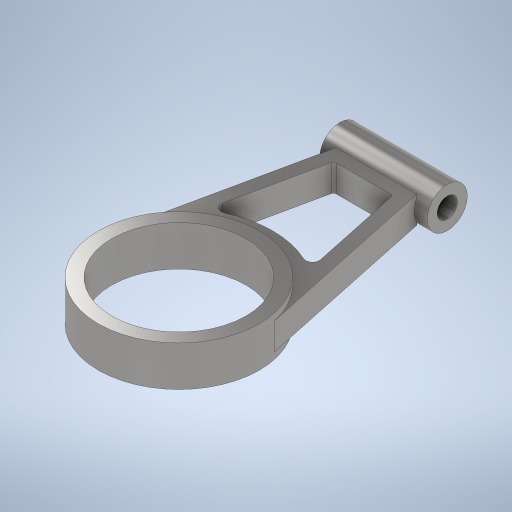
# Autodesk Inventor part: Excercise4
Saved by Autodesk Inventor 2024 (Build 280153000, 153)
## iProperties
Created: 2024-03-22
Part Number: Excercise4
Material: Stahl, galvanisiert
Document SubType Name: Modeling
Designer: ffogue
Density: 7.85 g/cm^3
Appearance: Galvanisiert
Author: ffogue
Autodesk Inventor part; units mm, degrees
ref_plane "XZ Plane" through (0, 0, 0) normal (0, 1, 0) x (-1, 0, 0)
ref_plane "XY Plane" through (0, 0, 0) normal (0, 0, 1) x (1, 0, 0)
sketch "Skizze1" plane through (0, 0, 0) normal (0, 0, 1) x (1, 0, 0)
  circle A0 centre (0, 0) radius 60
  line L0 (-58.6889, 12.4747) -> (-30, 147.4452)
  line L1 (58.6889, 12.4747) -> (30, 147.4452)
  line L2 (30, 147.4452) -> (-30, 147.4452)
  line L3 (0, 0) -> (0, 147.4452) construction
  dimension "d0" = 120
  dimension "d1" = 24
  dimension "d2" = 60
  constraints: 8 end point, 2 point on circle, 2 tangent, 1 centre point, 1 coincident, 1 horizontal, 1 midpoint, 1 symmetric about line, 1 vertical
  measures "d0" diameter of A0
  measures "d1" angle of L1 L0
  measures "d2" distance of L1.end L0.end
extrude "Extrusion1" add sketch "Skizze1" along normal mid plane 30 contours A0
extrude "Extrusion2" add sketch "Skizze1" along normal mid plane 20 contours A0 L0 L2 L1
sketch "Skizze2" plane through (0, 0, 15) normal (0, 0, 1) x (1, 0, 0)
  circle A0 centre (0, 0) radius 50
  dimension "d7" = 100
  constraints: 1 centre point, 1 coincident
  measures "d7" diameter of A0
extrude "Extrusion3" cut sketch "Skizze2" against normal up to surface (30 mm away)
ref_plane "Arbeitsebene1" through (0, 0, 0) normal (1, 0, 0) x (0, 1, 0)
sketch "Skizze3" plane through (0, 0, 0) normal (1, 0, 0) x (0, 1, 0)
  line L0 (147.4452, 10) -> (12.4747, 10) projected
  line L1 (12.4747, 10) -> (12.4747, 10) projected
  line L2 (12.4747, 10) -> (147.4452, 10) projected
  circle A0 centre (160, 0) radius 15
  circle A1 centre (160, 0) radius 7.5
  point P0 (0, 0)
  dimension "d11" = 30
  dimension "d12" = 160
  dimension "d13" = 15
  constraints: 2 centre point, 1 coincident, 1 horizontal alignment
  measures "d11" diameter of A0
  measures "d12" distance of point (0, 0) A0.centre
  measures "d13" diameter of A1
extrude "Extrusion4" add sketch "Skizze3" along normal mid plane 80
sketch "Skizze4" plane through (0, 0, 10) normal (0, 0, 1) x (1, 0, 0)
  line L0 (-21.9022, 137.4452) -> (21.9022, 137.4452)
  line L1 (21.9022, 137.4452) -> (38.7218, 58.3148)
  line L2 (-38.7218, 58.3148) -> (-21.9022, 137.4452)
  line L3 (0, 0) -> (0, 147.2716) construction
  line L4 (-30, 147.4452) -> (-58.6889, 12.4747) projected
  line L5 (58.6889, 12.4747) -> (30, 147.4452) projected
  line L6 (30, 147.4452) -> (-30, 147.4452) projected
  arc A0 (38.7218, 58.3148) -> (-38.7218, 58.3148) centre (0, 0) ccw
  circle A1 centre (0, 0) radius 60 projected
  dimension "d16" = 10
  dimension "d17" = 10
  dimension "d18" = 70
  constraints: 8 end point, 3 parallel, 2 point on circle, 2 symmetric about line, 1 centre point, 1 concentric, 1 horizontal, 1 vertical
  measures "d16" distance between parallel lines of L2 L4
  measures "d17" distance between parallel lines of L0 L6
  measures "d18" radius of A0
extrude "Extrusion5" cut sketch "Skizze4" against normal up to surface (20 mm away) contours L0 L1 A0 L2
fillet "Rundung1" radius 5 2 edges at (-38.7218, 58.3148, 0) (38.7218, 58.3148, 0)
fillet "Rundung2" radius 2 2 edges at (21.9022, 137.4452, 0) (-21.9022, 137.4452, 0)
